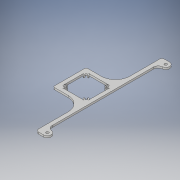
# Autodesk Inventor part: CameraBracket
Saved by Autodesk Inventor 2018 (Build 220112000, 112)
## iProperties
Created: 2019-10-25
Part Number: CameraBracket
Material: Generic
Document SubType Name: Modeling
Designer: anirudh
Density: 1 g/cm^3
Appearance: Default
Author: anirudh
Autodesk Inventor part; units mm, degrees
ref_plane "YZ Plane" through (0, 0, 0) normal (1, 0, 0) x (0, 1, 0)
ref_plane "XZ Plane" through (0, 0, 0) normal (0, 1, 0) x (-1, 0, 0)
ref_plane "XY Plane" through (0, 0, 0) normal (0, 0, 1) x (1, 0, 0)
sketch "Sketch1" plane through (0, 0, 0) normal (0, 1, 0) x (-1, 0, 0)
  circle A0 centre (-5.08, 6.35) radius 1.75
  circle A1 centre (-5.08, 6.35) radius 1.75
  arc A2 (-5.08, 11.43) -> (-5.08, 1.27) centre (-5.08, 6.35) ccw
  line L0 (0, 11.43) -> (0, 59.8834)
  line L1 (-5.08, 1.27) -> (5.0316, 1.27)
  line L2 (5.0316, 1.27) -> (5.0316, 63.0584)
  line L3 (-5.08, 11.43) -> (0, 11.43)
  line L4 (0, 11.43) -> (0, 59.8834)
  line L5 (5.0316, 63.0584) -> (42.3132, 63.0584)
  line L6 (5.0316, 63.0584) -> (42.3132, 63.0584)
  line L7 (44.0632, 64.8084) -> (44.0632, 105.3716)
  line L8 (44.0632, 64.8084) -> (44.0632, 105.3716)
  line L9 (42.3132, 107.1216) -> (5.0316, 107.1216)
  line L10 (42.3132, 107.1216) -> (5.0316, 107.1216)
  line L11 (5.0316, 107.1216) -> (5.0316, 168.91)
  circle A3 centre (-5.08, 163.83) radius 1.75
  circle A4 centre (-5.08, 163.83) radius 1.75
  arc A5 (-5.08, 168.91) -> (-5.08, 158.75) centre (-5.08, 163.83) ccw
  line L12 (0, 110.2966) -> (0, 158.75)
  line L13 (-5.08, 168.91) -> (5.0316, 168.91)
  line L14 (0, 59.8834) -> (0, 158.75)
  line L15 (0, 158.75) -> (-5.08, 158.75)
  arc A6 (8.0362, 72.5946) -> (9.5362, 71.0946) centre (8.0362, 71.0946) ccw
  arc A7 (8.0362, 72.5946) -> (9.5362, 71.0946) centre (8.0362, 71.0946) ccw
  arc A8 (34.527, 71.0946) -> (36.027, 72.5946) centre (36.027, 71.0946) ccw
  arc A9 (34.527, 71.0946) -> (36.027, 72.5946) centre (36.027, 71.0946) ccw
  arc A10 (36.027, 97.5854) -> (34.527, 99.0854) centre (36.027, 99.0854) ccw
  arc A11 (36.027, 97.5854) -> (34.527, 99.0854) centre (36.027, 99.0854) ccw
  arc A12 (9.5362, 99.0854) -> (8.0362, 97.5854) centre (8.0362, 99.0854) ccw
  arc A13 (9.5362, 99.0854) -> (8.0362, 97.5854) centre (8.0362, 99.0854) ccw
  arc A14 (8.0362, 68.09) -> (11.0408, 71.0946) centre (8.0362, 71.0946) ccw
  arc A15 (33.0224, 71.0946) -> (36.027, 68.09) centre (36.027, 71.0946) ccw
  line L16 (11.0408, 99.0854) -> (9.5362, 99.0854)
  line L17 (36.027, 68.09) -> (8.0362, 68.09)
  line L18 (8.0362, 68.09) -> (36.027, 68.09)
  line L19 (5.0316, 99.0854) -> (5.0316, 71.0946)
  line L20 (5.0316, 71.0946) -> (5.0316, 99.0854)
  line L21 (8.0362, 102.09) -> (36.027, 102.09)
  line L22 (8.0362, 102.09) -> (36.027, 102.09)
  line L23 (39.0316, 71.0946) -> (39.0316, 99.0854)
  line L24 (39.0316, 71.0946) -> (39.0316, 99.0854)
  line L25 (33.0224, 71.0946) -> (34.527, 71.0946)
  line L26 (34.527, 71.0946) -> (33.0224, 71.0946)
  line L27 (36.027, 72.5946) -> (36.027, 74.0992)
  line L28 (36.027, 72.5946) -> (36.027, 74.0992)
  line L29 (9.5362, 71.0946) -> (11.0408, 71.0946)
  line L30 (11.0408, 71.0946) -> (9.5362, 71.0946)
  line L31 (8.0362, 74.0992) -> (8.0362, 72.5946)
  line L32 (8.0362, 72.5946) -> (8.0362, 74.0992)
  line L33 (8.0362, 96.0808) -> (8.0362, 97.5854)
  line L34 (8.0362, 96.0808) -> (8.0362, 97.5854)
  arc A16 (11.0408, 99.0854) -> (8.0362, 102.09) centre (8.0362, 99.0854) ccw
  line L35 (9.5362, 99.0854) -> (11.0408, 99.0854)
  line L36 (36.027, 97.5854) -> (36.027, 96.0808)
  line L37 (36.027, 96.0808) -> (36.027, 97.5854)
  line L38 (33.0224, 99.0854) -> (34.527, 99.0854)
  line L39 (34.527, 99.0854) -> (33.0224, 99.0854)
  arc A17 (36.027, 96.0808) -> (39.0316, 99.0854) centre (36.027, 99.0854) ccw
  arc A18 (36.027, 102.09) -> (33.0224, 99.0854) centre (36.027, 99.0854) ccw
  arc A19 (33.0224, 71.0946) -> (36.027, 68.09) centre (36.027, 71.0946) ccw
  arc A20 (39.0316, 71.0946) -> (36.027, 74.0992) centre (36.027, 71.0946) ccw
  arc A21 (8.0362, 68.09) -> (11.0408, 71.0946) centre (8.0362, 71.0946) ccw
  arc A22 (8.0362, 74.0992) -> (5.0316, 71.0946) centre (8.0362, 71.0946) ccw
  arc A23 (11.0408, 99.0854) -> (8.0362, 102.09) centre (8.0362, 99.0854) ccw
  arc A24 (5.0316, 99.0854) -> (8.0362, 96.0808) centre (8.0362, 99.0854) ccw
  arc A25 (44.0632, 105.3716) -> (42.3132, 107.1216) centre (42.3132, 105.3716) ccw
  arc A26 (42.3132, 63.0584) -> (44.0632, 64.8084) centre (42.3132, 64.8084) ccw
  point P0 (0, 0)
  point P1 (0, 0)
  point P2 (3.175, 59.8834)
  constraints: 80 end point, 46 point on circle, 27 centre point, 12 coincident, 10 collinear, 6 tangent, 4 horizontal, 4 perpendicular, 4 vertical
extrude "Extrusion1" add sketch "Sketch1" along normal blind 2.54
fillet "Fillet1" radius 6.35 2 edges at (0, 1.27, 11.43) (0, 1.27, 158.75)
fillet "Fillet2" radius 3.175 2 edges at (-5.0316, 1.27, 1.27) (-5.0316, 1.27, 168.91)
fillet "Fillet3" radius 19.05 2 edges at (-5.0316, 1.27, 107.1216) (-5.0316, 1.27, 63.0584)
body "Solid1"
